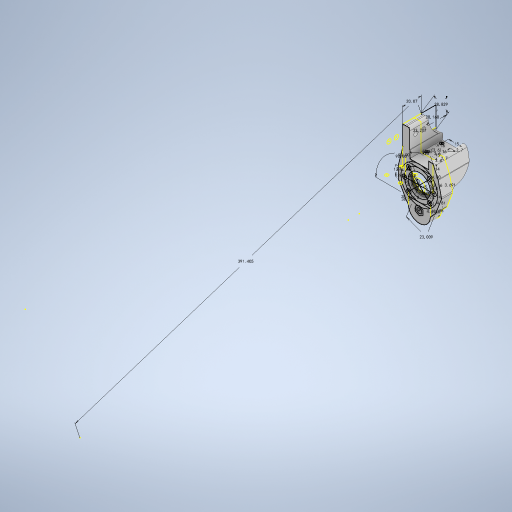
# Autodesk Inventor part: 零件2591
Saved by Autodesk Inventor 2023.1 (Build 271208000, 208)
## iProperties
Created: 2022-09-11
Part Number: 零件2591
Material: 常规
Document SubType Name: Modeling
Designer: yao19
Density: 1 g/cm^3
Appearance: 默认
Author: yao19
## iProperties of the stored document 零件2591_3D 打印.ipt
Created: 2022-09-11
Part Number: 零件2591_3D 打印
Material: 常规
Document SubType Name: Modeling
Designer: yao19
Density: 1 g/cm^3
Appearance: 默认
Author: yao19
Autodesk Inventor part; units mm, degrees
ref_plane "YZ Plane" through (0, 0, 0) normal (1, 0, 0) x (0, 1, 0)
ref_plane "XZ Plane" through (0, 0, 0) normal (0, 1, 0) x (-1, 0, 0)
ref_plane "XY Plane" through (0, 0, 0) normal (0, 0, 1) x (1, 0, 0)
sketch "草图3" plane through (62.6992, 71.6899, -352.2266) normal (0, 0, -1) x (-1, 0, 0)
  circle A0 centre (-14.7011, -0.0006) radius 6.4013 projected
  line L0 (-14.7, -28.8497) -> (-12, -27.2909) projected
  line L1 (-17.4, -27.2909) -> (-14.7, -28.8497) projected
  line L2 (-4.4962, 19.8985) -> (-24.8962, 19.8985) projected
  line L3 (-4.4962, 27.8985) -> (-4.4962, 19.8985) projected
  circle A1 centre (-14.7011, -0.0006) radius 20
  circle A2 centre (-14.7011, -0.0006) radius 16.1
  circle A3 centre (-14.7011, -0.0006) radius 12.1
  line L4 (-2.8357, 16.0994) -> (-26.5666, 16.0994)
  line L5 (-2.8357, -16.1006) -> (-26.5666, -16.1006)
  line L6 (-14.7011, -0.0006) -> (-3.3167, 11.3839)
  line L7 (-14.7011, -0.0006) -> (1.3989, -0.0006)
  line L8 (-14.7011, -0.0006) -> (-3.3167, -11.385)
  line L9 (-14.7011, -0.0006) -> (-30.8011, -0.0006)
  line L10 (-14.7011, -0.0006) -> (-26.0856, 11.3839)
  line L11 (-14.7011, -0.0006) -> (-26.0856, -11.385)
  circle A4 centre (1.3989, -0.0006) radius 2.4
  circle A5 centre (-3.3167, 11.3839) radius 2.4
  circle A6 centre (-3.3167, -11.385) radius 2.4
  line L12 (-4.1962, 28.1985) -> (-4.4962, 27.8985) projected
  line L13 (-4.1962, 48.8985) -> (-4.1962, 28.1985) projected
  line L14 (2.3038, 48.8985) -> (-4.1962, 48.8985) projected
  line L15 (3.3038, 28.1653) -> (3.3038, 47.8985) projected
  line L16 (0.4, 0) -> (0.4, 18.8433) projected
  line L17 (-2.7, -24) -> (-2.7, -12.0835) projected
  line L18 (-26.7, -12.0835) -> (-26.7, -24) projected
  line L19 (-24.8962, 19.8985) -> (-24.8962, 27.8985) projected
  line L20 (-24.8962, 27.8985) -> (-28.8, 27.8985) projected
  line L21 (-29.8, 26.8985) -> (-29.8, 0) projected
  line L22 (-4.4962, 19.8985) -> (-4.4962, 27.8985)
  line L23 (-4.1962, 28.1985) -> (-4.1962, 48.8985)
  line L24 (-4.4962, 27.8985) -> (-4.1962, 28.1985)
  line L25 (-4.1962, 48.8985) -> (2.3038, 48.8985)
  line L26 (2.3038, 48.8985) -> (3.3038, 48.8985)
  line L27 (3.3038, 48.8985) -> (3.3038, 28.1653)
  line L28 (3.2127, 27.6477) -> (8.2989, 6.9731)
  line L29 (8.2989, 6.9731) -> (8.2989, -5.0269)
  line L30 (8.2989, -5.0269) -> (-0.0087, -20.3677)
  line L31 (-0.0087, -20.3677) -> (-2.7, -24)
  line L32 (-4.4962, 19.8985) -> (-24.8962, 19.8985)
  line L33 (-24.8962, 27.8985) -> (-24.8962, 19.8985)
  line L34 (-24.8962, 27.8985) -> (-29.6456, 27.8985)
  line L35 (-29.6456, 27.8985) -> (-35.3399, 15.1089)
  line L36 (-35.3399, 15.1089) -> (-39.0383, -0.7028)
  line L37 (-39.0383, -0.7028) -> (-32.6645, -17.5366)
  line L38 (-32.6645, -17.5366) -> (-26.7, -24)
  arc A7 (-26.7, -24) -> (-2.7, -24) centre (-14.7, -24) ccw
  circle A8 centre (-14.7, -24) radius 2.7
  line L39 (-14.7, -28.8497) -> (-18.9, -26.4249)
  line L40 (-18.9, -26.4249) -> (-18.9, -21.5751)
  line L41 (-18.9, -21.5751) -> (-14.7, -19.1503)
  line L42 (-14.7, -19.1503) -> (-10.5, -21.5751)
  line L43 (-10.5, -21.5751) -> (-10.5, -26.4249)
  line L44 (-10.5, -26.4249) -> (-14.7, -28.8497)
  line L45 (3.3038, 28.1653) -> (3.2127, 27.6477)
  circle A9 centre (-26.0856, 11.3839) radius 2.4
  circle A10 centre (-30.8011, -0.0006) radius 2.4
  circle A11 centre (-26.0856, -11.385) radius 2.4
  point P0 (62.6992, -71.6899)
  dimension "d18" = 32.2
  dimension "d17" = 40
  dimension "d19" = 24.2
  dimension "d20" = 90
  dimension "d21" = 90
  dimension "d22" = 45
  dimension "d23" = 45
  dimension "d24" = 45
  dimension "d25" = 45
  dimension "d26" = 4.8
  dimension "d27" = 4.8
  dimension "d28" = 4.8
  dimension "d33" = 24
  dimension "d35" = 12
  dimension "d36" = 23
  dimension "d37" = 24
  dimension "d38" = 28.437
  dimension "d39" = 36.536
  dimension "d40" = 14
  dimension "d41" = 25
  dimension "d42" = 13.165
  dimension "d43" = 20.738
  dimension "d44" = 18
  dimension "d45" = 23.0089
  dimension "d51" = 4.8
  dimension "d52" = 4.8
  dimension "d53" = 4.8
  dimension "d54" = 4.1011
  dimension "d57" = 5.4001
  constraints: 64 end point, 11 coincident, 10 centre point, 6 point on circle, 4 collinear, 3 horizontal, 3 point on line, 2 tangent, 2 vertical, 1 perpendicular, 22 other
  measures "d17" diameter of A1
  measures "d19" diameter of A3
  measures "d20" angle of L3 L4
  measures "d21" angle of L3 L5
  measures "d22" angle of L7 L6
  measures "d23" angle of L8 L7
  measures "d24" angle of L9 L10
  measures "d25" angle of L11 L9
  measures "d26" diameter of A4
  measures "d27" diameter of A5
  measures "d28" diameter of A6
  measures "d33" angle of L21 L35
  measures "d35" distance of L28.end L29.end
  measures "d36" distance from line of A1.centre L29
  measures "d37" distance from line of A1.centre L28
  measures "d38" angle of L17 L30
  measures "d39" angle of L17 L31
  measures "d40" distance of L34.end L35.end
  measures "d41" distance from line of A0.centre L35
  measures "d42" angle of L21 L36
  measures "d43" angle of L21 L37
  measures "d44" distance of L36.end L37.end
  measures "d45" distance from line of A0.centre L37
  measures "d51" diameter of A9
  measures "d52" diameter of A10
  measures "d53" diameter of A11
  measures "d54" distance from line of L18 A10.centre
  measures "d57" diameter of A8
extrude "拉伸1" add sketch "草图3" along normal blind 12.2 contours L4 A1 L2 | L5 A1 L42 L41 | A1 L2 L3 L12 L13 L14 L26 L27 L15 L45 L28 L29 L30 L31 L17 | A1 L18 L38 L37 L36 L35 L34 L20 L19 L2 | A1 L17 A7 L18 L41 L40 L39 L1 L0 L44 L43 L42 | L42 L43 L44 L0 L1 L39 L40 L41 A1 | A1 L41 L42 | A8
extrude "拉伸2" add sketch "草图3" along normal blind 3 contours L7 L6 A0 | L7 A3 L8 A0 | A0 L8 L7 | A0 L6 A3 L7 | L6 L10 A0 | A0 L10 A3 L6 | L8 A3 L11 A0 | A0 L11 L8 | L11 A0 L9 | L9 A0 L10 | L7 A4 A2 A6 L8 A3 | A3 L6 A5 A2 L16 A4 L7 | A0 L9 A3 L10 | A3 L10 A9 A2 A5 L6 | L11 A3 L9 A0 | L8 A6 A2 A11 L11 A3 | A3 L9 A10 L21 A2 A9 L10 | L11 A11 A2 A10 L9 A3 | L16 A2 A4 | A4 A2 L16 A1 L17 A6 | A9 A2 L10 | L10 A2 A9 | A2 L4 A1 L16 A5 | A11 A2 L11 | L11 A2 A11 | A6 L17 A1 L5 A2 | A10 A2 L9 | L9 L21 A10 | A2 A9 | A2 L21 A1 L4 A9 | A2 A11 | A11 L18 A1 L21 A2 A10 | L5 A1 L18 A11 A2 | L9 A2 A10 L21 | A10 A2 L21 | A10 A2
extrude "拉伸3" cut sketch "草图3" along normal through all contours L7 L6 A0 | L7 A3 L8 A0 | A0 L8 L7 | A0 L6 A3 L7 | L6 L10 A0 | A0 L10 A3 L6 | L8 A3 L11 A0 | A0 L11 L8 | L11 A0 L9 | L9 A0 L10 | A0 L9 A3 L10 | L11 A3 L9 A0 | A9 A2 L10 | L10 A2 A9 | A11 A2 L11 | L11 A2 A11 | A10 A2 L9 | L9 L21 A10 | A2 A9 | A2 A11 | L9 A2 A10 L21 | A10 A2
extrude "拉伸4" cut sketch "草图3" along normal blind 4 contours L42 L43 L44 L0 L1 L39 L40 L41 A1 | A1 L41 L42 | A8
sketch "草图4" plane through (62.6992, 71.6899, -364.4266) normal (0, 0, -1) x (-1, 0, 0)
  circle A0 centre (-14.7, -24) radius 2.7 projected
  circle A1 centre (-14.7, -24) radius 4.5
  arc A2 (-26.5666, 16.0994) -> (-26.5666, -16.1006) centre (-14.7011, -0.0006) ccw projected
  line L0 (-34.4632, 3.0756) -> (-38.1545, 3.0756)
  line L1 (-35.3399, 15.1089) -> (-39.0383, -0.7028) projected
  arc A3 (-2.8357, -16.1006) -> (-2.8357, 16.0994) centre (-14.7011, -0.0006) ccw projected
  line L2 (5.0609, 3.0756) -> (8.2989, 3.0756)
  line L3 (8.2989, -5.0269) -> (8.2989, 6.9731) projected
  line L4 (-24.8962, 19.8985) -> (-24.8962, 27.8985) projected
  line L5 (-24.8962, 27.8985) -> (-29.6456, 27.8985) projected
  line L6 (-29.6456, 27.8985) -> (-35.3399, 15.1089) projected
  line L7 (-35.3399, 15.1089) -> (-39.0383, -0.7028) projected
  line L8 (-39.0383, -0.7028) -> (-32.6645, -17.5366) projected
  line L9 (-32.6645, -17.5366) -> (-26.7, -24) projected
  arc A4 (-26.7, -24) -> (-2.7, -24) centre (-14.7, -24) ccw projected
  line L10 (-2.7, -24) -> (-0.0087, -20.3677) projected
  line L11 (-0.0087, -20.3677) -> (8.2989, -5.0269) projected
  line L12 (8.2989, -5.0269) -> (8.2989, 6.9731) projected
  line L13 (8.2989, 6.9731) -> (3.2127, 27.6477) projected
  line L14 (3.2127, 27.6477) -> (3.3038, 28.1653) projected
  line L15 (3.3038, 28.1653) -> (3.3038, 48.8985) projected
  line L16 (3.3038, 48.8985) -> (-4.1962, 48.8985) projected
  line L17 (-4.1962, 48.8985) -> (-4.1962, 28.1985) projected
  line L18 (-4.1962, 28.1985) -> (-4.4962, 27.8985) projected
  line L19 (-4.4962, 27.8985) -> (-4.4962, 19.8985) projected
  line L20 (-4.4962, 19.8985) -> (-24.8962, 19.8985) projected
  arc A5 (-2.8357, -16.1006) -> (-2.8357, 16.0994) centre (-14.7011, -0.0006) ccw projected
  line L21 (-2.8357, -16.1006) -> (-26.5666, -16.1006) projected
  arc A6 (-26.5666, 16.0994) -> (-26.5666, -16.1006) centre (-14.7011, -0.0006) ccw projected
  line L22 (-26.5666, 16.0994) -> (-2.8357, 16.0994) projected
  point P0 (62.6992, -71.6899)
  dimension "d62" = 9
  dimension "d63" = 3.6913
  constraints: 4 end point, 4 point on line, 2 point on circle, 1 centre point, 1 coincident, 1 horizontal
  measures "d62" diameter of A1
  measures "d63" distance of L0.start L0.end
extrude "拉伸6" add sketch "草图4" along normal blind 4 contours A1
extrude "拉伸7" add sketch "草图4" along normal blind 24 contours A2 L0 L1 L6 L5 L4 L20 L19 L18 L17 L16 L15 L14 L13 L3 L2 A3 L22
sketch "草图5" plane through (67.1954, 91.5884, -352.2266) normal (0, 1, 0) x (1, 0, 0)
  circle A0 centre (2.7007, -11.951) radius 1.7988 projected
  circle A1 centre (17.7006, -11.9508) radius 1.7991 projected
  circle A2 centre (17.7003, -27.9506) radius 1.7994 projected
  circle A3 centre (2.6988, -27.949) radius 1.8016 projected
  line L0 (0, 0) -> (20.4, 0) projected
  line L1 (20.4, 0) -> (0, 0)
  circle A4 centre (2.7007, 11.951) radius 1.7988 construction
  circle A5 centre (17.7006, 11.9508) radius 1.7991 construction
  circle A6 centre (17.7003, 27.9506) radius 1.7994 construction
  circle A7 centre (2.6988, 27.949) radius 1.8016 construction
  circle A8 centre (17.7005, 15.9508) radius 1.8
  circle A9 centre (17.7003, 31.9508) radius 1.8
  line L2 (20.4, 0) -> (20.4, 36.2) projected
  circle A10 centre (2.7005, 15.951) radius 1.8
  circle A11 centre (2.7003, 31.951) radius 1.8
  point P0 (-67.1954, -352.2266)
  dimension "d86" = 3.6
  dimension "d87" = 3.6
  dimension "d88" = 4
  dimension "d89" = 2.6995
  dimension "d90" = 16
  dimension "d91" = 2.6997
  dimension "d92" = 3.6
  dimension "d93" = 3.6
  dimension "d94" = 16
  dimension "d95" = 4
  dimension "d96" = 15
  dimension "d97" = 15
  constraints: 8 centre point, 4 symmetric about line, 2 end point, 2 equal radius, 1 collinear, 4 other
  measures "d86" diameter of A8
  measures "d87" diameter of A9
  measures "d88" distance of A5.centre A8.centre
  measures "d89" distance from line of L2 A8.centre
  measures "d90" distance of A8.centre A9.centre
  measures "d91" distance from line of L2 A9.centre
  measures "d92" diameter of A10
  measures "d93" diameter of A11
  measures "d94" distance of A11.centre A10.centre
  measures "d95" distance of A4.centre A10.centre
  measures "d96" distance of A8.centre A10.centre
  measures "d97" distance of A9.centre A11.centre
extrude "拉伸8" cut sketch "草图5" against normal through all contours A8 | A9 | A10 | A11
extrude "拉伸9" cut sketch "草图3" along normal through all contours A8
fillet "圆角2" radius 3 12 edges at (101.7375, 70.9871, -358.3266) (98.0391, 86.7988, -370.3266) (89.3992, 47.6899, -358.3266) (65.3992, 47.6899, -358.3266) (62.7079, 51.3222, -358.3266) (54.4004, 66.663, -358.3266) (54.4004, 78.663, -370.3266) (59.3954, 120.5884, -370.3266) (66.8954, 120.5884, -370.3266) (92.3448, 99.5884, -370.3266) (87.5954, 99.5884, -370.3266) (95.3637, 54.1534, -358.3266)
fillet "圆角3" radius 22 1 edges at (99.0081, 74.7655, -388.4266)
fillet "圆角4" radius 4 2 edges at (99.0081, 74.7655, -364.4266) (56.0194, 74.7655, -364.4266)
sketch "草图6" plane through (59.3954, 99.8552, -388.4266) normal (-1, 0, 0) x (0, 0, 1)
  circle A0 centre (43.1997, 11.7328) radius 2.3495 projected
  circle A1 centre (51.1988, 11.7314) radius 2.3479 projected
  line L0 (36.2, 0) -> (36.2, 19.7332) projected
  line L1 (36.2, 0) -> (36.2, 17.7332) projected
  line L2 (36.2, 0) -> (36.2, 17.7332)
  circle A2 centre (29.2003, 11.7328) radius 2.3495
  circle A3 centre (21.2012, 11.7314) radius 2.3479
  arc A4 (0.2067, -3.0897) -> (16.1295, 20.9436) centre (-12.006, 22.2929) ccw
  line L3 (36.2, 20.7332) -> (0, 20.7332) projected
  line L4 (16.1186, 20.7332) -> (0, 20.7332)
  arc A5 (0, -3.0897) -> (9.0016, -20.8391) centre (22, -3.0897) ccw projected
  line L5 (36.2, -20.8391) -> (9.0016, -20.8391) projected
  line L6 (36.2, -20.8391) -> (36.2, -0.5176) projected
  line L7 (36.2, -0.5176) -> (0, -0.5176) projected
  line L8 (0, -3.0897) -> (0, -0.5176) projected
  line L9 (0, -3.0897) -> (0, -0.5176) projected
  line L10 (0, -3.0897) -> (0, 20.7332)
  point P0 (388.4266, -99.8552)
  point P1 (4.52, -0.5176)
  dimension "d78" = 28.1678
  dimension "d79" = 33.2072
  dimension "d80" = 28.8295
  dimension "d81" = 20.0705
  dimension "d82" = 391.4045
  constraints: 6 end point, 3 centre point, 3 point on circle, 2 collinear, 2 symmetric about line, 1 point on line, 1 vertical, 2 other
  measures "d78" radius of A4
  measures "d79" horizontal distance of A3.centre A4.centre
  measures "d80" distance of A4.start A4.end
  measures "d81" distance from line of A4.end L0
  measures "d82" distance of point (388.427, -99.855) A4.end
extrude "拉伸10" cut sketch "草图6" against normal through all contours A2 | A3
extrude "拉伸11" cut sketch "草图6" against normal blind 10 contours L7 L10 L3 A4
fillet "圆角5" radius 3 1 edges at (63.341, 99.3376, -388.4266)
fillet "圆角6" radius 4 1 edges at (81.8992, 47.6899, -364.4266)
